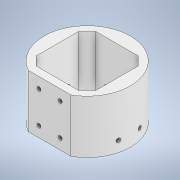
# Autodesk Inventor part: brazo_articulado_2
Saved by Autodesk Inventor 2021 (Build 250183000, 183)
## iProperties
Created: 2021-04-15
Part Number: brazo_articulado_2
Material: Plástico ABS
Document SubType Name: Modeling
Designer: Joaquín
Density: 1.06 g/cm^3
Appearance: Suave - Blanco
Author: Joaquín
Autodesk Inventor part; units mm, degrees
ref_plane "YZ Plane" through (0, 0, 0) normal (1, 0, 0) x (0, 1, 0)
ref_plane "XZ Plane" through (0, 0, 0) normal (0, 1, 0) x (-1, 0, 0)
ref_plane "XY Plane" through (0, 0, 0) normal (0, 0, 1) x (1, 0, 0)
sketch "Boceto1" plane through (0, 0, 0) normal (0, 1, 0) x (-1, 0, 0)
  circle A0 centre (0, 0) radius 32.5
  line L0 (0, -22.5) -> (16, -22.5)
  line L1 (0, -22.5) -> (-16, -22.5)
  line L2 (-22.5, 0) -> (-22.5, -16)
  line L3 (-22.5, 0) -> (-22.5, 16)
  line L4 (0, 22.5) -> (16, 22.5)
  line L5 (0, 22.5) -> (-16, 22.5)
  line L6 (-16, 22.5) -> (-22.5, 16)
  line L7 (-22.5, -16) -> (-16, -22.5)
  line L8 (22.5, 0) -> (22.5, 16)
  line L9 (22.5, 0) -> (22.5, -16)
  line L10 (22.5, -16) -> (16, -22.5)
  line L11 (16, 22.5) -> (22.5, 16)
  constraints: 24 end point, 4 horizontal, 4 vertical, 1 centre point, 1 point on line
extrude "Extrusión1" add sketch "Boceto1" along normal blind 40
sketch "Boceto14" plane through (0, 0, 0) normal (0, -1, 0) x (1, 0, 0)
  line L0 (-16, 28.2887) -> (16, 28.2887)
  arc A0 (16, 28.2887) -> (-16, 28.2887) centre (0, 0) ccw
  point P0 (16, 22.5)
  point P1 (-16, 22.5)
  constraints: 2 end point, 2 point on circle, 1 centre point, 1 coincident, 1 horizontal
extrude "Extrusión10" cut sketch "Boceto14" against normal blind 40
sketch "Boceto15" plane through (-22.5, 0, 16) normal (1, 0, 0) x (0, 0, -1)
  circle A0 centre (8, 8) radius 1.5
  circle A1 centre (24, 8) radius 1.5
  point P0 (16, 0)
  point P1 (0, 0)
  dimension "d80" = 3
  dimension "d81" = 3
  constraints: 2 centre point
  measures "d80" diameter of A0
  measures "d81" diameter of A1
extrude "Extrusión11" cut sketch "Boceto15" against normal mid plane 200
sketch "Boceto16" plane through (16, 0, 22.5) normal (0, 0, -1) x (-1, 0, 0)
  line L0 (-6.5, 0) -> (0, 0) projected
  circle A0 centre (8, 8) radius 1.5
  circle A1 centre (24, 8) radius 1.5
  point P0 (16, 0)
  dimension "d88" = 3
  dimension "d89" = 3
  constraints: 2 centre point
  measures "d88" diameter of A0
  measures "d89" diameter of A1
extrude "Extrusión12" cut sketch "Boceto16" along normal mid plane 200
sketch "Boceto17" plane through (16, 0, 22.5) normal (0, 0, -1) x (-1, 0, 0)
  circle A0 centre (8, 32) radius 1.5
  circle A1 centre (24, 32) radius 1.5
  point P0 (16, 0)
  point P1 (0, 40)
  dimension "d95" = 3
  dimension "d96" = 3
  constraints: 2 centre point
  measures "d95" diameter of A0
  measures "d96" diameter of A1
extrude "Extrusión13" cut sketch "Boceto17" against normal blind 200
